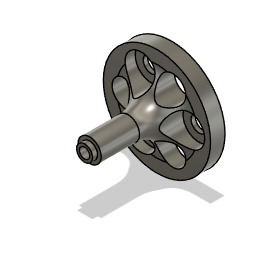
hangfa-discovery-q2_optitrack_wheels-trackers_support (Autodesk Fusion 360 design; units mm, degrees)
Autodesk Fusion 360 part; units mm, degrees
sketch "Sketch1" plane through (0, 0, 0) normal (0, 0, 1) x (1, 0, 0)
  circle A0 centre (0, 0) radius 11 construction
  circle A1 centre (11, 0) radius 2.75
  circle A2 centre (5.5, 9.5263) radius 2.75 construction
  circle A3 centre (-5.5, 9.5263) radius 2.75
  circle A4 centre (-11, 0) radius 2.75 construction
  circle A5 centre (-5.5, -9.5263) radius 2.75
  circle A6 centre (5.5, -9.5263) radius 2.75 construction
  circle A7 centre (0, 0) radius 1.8
  line L0 (0, 0) -> (11, 0) construction
  circle A8 centre (11, 0) radius 5.5 construction
  circle A9 centre (0, 0) radius 16.5 construction
  circle A10 centre (0, 0) radius 18.5
  circle A11 centre (5.5, 9.5263) radius 4.5
  circle A12 centre (-11, 0) radius 4.5
  circle A13 centre (5.5, -9.5263) radius 4.5
  dimension "d1" = 5.5
  dimension "d2" = 22
  dimension "d4" = 360
  dimension "d6" = 3.6
  dimension "d8" = 11
  dimension "d9" = 2
  dimension "d12" = 9
  constraint coincident A0.centre A7.centre
  constraint concentric A0 A7
  constraint coincident A0 A1.centre
  constraint coincident A1.centre L0.end
  constraint horizontal L0
  constraint concentric A1 A8
  constraint tangent A8 A9
  constraint concentric A2 A11
  constraint concentric A4 A12
  constraint concentric A6 A13
  constraint equal A11 A12
  constraint equal A11 A13
  measures "d1" diameter of A1
  measures "d2" diameter of A0
  measures "d6" diameter of A7
  measures "d8" diameter of A8
  measures "d12" diameter of A11
extrude "Extrude1" add sketch "Sketch1" along normal blind 1.5
sketch "Sketch3" plane through (0, 0, 1.5) normal (0, 0, 1) x (1, 0, 0)
  circle A0 centre (0, 0) radius 1.8
  circle A1 centre (-11, 0) radius 4.5
  circle A2 centre (11, 0) radius 2.75
  circle A3 centre (-5.5, -9.5263) radius 2.75
  circle A4 centre (-5.5, 9.5263) radius 2.75
  circle A5 centre (5.5, -9.5263) radius 4.5
  circle A6 centre (5.5, 9.5263) radius 4.5
  circle A7 centre (0, 0) radius 18.5
  circle A8 centre (-5.5, 9.5263) radius 5.5
  circle A9 centre (11, 0) radius 5.5
  circle A10 centre (-5.5, -9.5263) radius 5.5
  dimension "d13" = 11
  constraint concentric A4 A8
  constraint concentric A2 A9
  constraint concentric A3 A10
  constraint equal A8 A10
  constraint equal A8 A9
  measures "d13" diameter of A8
extrude "Extrude2" add sketch "Sketch3" along normal blind 3.5 contours A7
sketch "Sketch4" plane through (0, 0, 5) normal (0, 0, 1) x (1, 0, 0)
  circle A0 centre (-5.5, -9.5263) radius 5.5
  circle A1 centre (-5.5, 9.5263) radius 5.5
  circle A2 centre (5.5, 9.5263) radius 4.5
  circle A3 centre (5.5, -9.5263) radius 4.5
  circle A4 centre (-11, 0) radius 4.5
  circle A5 centre (0, 0) radius 1.8
  circle A6 centre (11, 0) radius 5.5
  circle A7 centre (0, 0) radius 18.5
  circle A8 centre (0, 0) radius 4
  dimension "d16" = 8
  constraint coincident A5.centre A7.centre
  measures "d16" diameter of A8
extrude "Extrude3" add sketch "Sketch4" along normal blind 25 contours A8
hole "Hole1" at (0, 0, 0) direction (0, 0, 1) diameter 3.5 depth 30 tip angle 180 countersink diameter 9 countersink angle 90
sketch "Sketch5" plane through (0, 0, 30) normal (0, 0, 1) x (1, 0, 0)
  circle A0 centre (0, 0) radius 1.8
  circle A1 centre (0, 0) radius 4
  circle A2 centre (0, 0) radius 2.75
  dimension "d24" = 5.5
  constraint coincident A0.centre A1.centre
  measures "d24" diameter of A2
extrude "Extrude4" cut sketch "Sketch5" against normal blind 1.75 contours A1
fillet "Fillet1" radius 10 1 edges at (-3.7293, 1.4465, 5)
